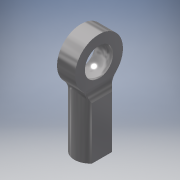
# Autodesk Inventor part: 10-32SuperDutyLinkage-1111-2017
Saved by Autodesk Inventor 2016 SP2 (Build 200236200, 236)
## iProperties
Created: 2017-02-16
Part Number: 10-32SuperDutyLinkage-1111-2017
Material: Stainless Steel
Document SubType Name: Modeling
Designer: 589013
Density: 8 g/cm^3
Appearance: Semi-Polished
Mass: 11.5391 g
Surface Area: 17.147 cm^2
Volume: 1.44239 cm^3
Author: 589013
Autodesk Inventor part; units mm, degrees
ref_plane "YZ Plane" through (0, 0, 0) normal (1, 0, 0) x (0, 1, 0)
ref_plane "XZ Plane" through (0, 0, 0) normal (0, 1, 0) x (-1, 0, 0)
ref_plane "XY Plane" through (0, 0, 0) normal (0, 0, 1) x (1, 0, 0)
sketch "Sketch1" plane through (0, 0, 0) normal (1, 0, 0) x (0, 1, 0)
  circle A0 centre (0, 0) radius 7.9375
  arc A1 (0, 5.55625) -> (0, -5.55625) centre (0, 0) ccw
  circle A2 centre (0, 0) radius 5.159375 construction
  line L0 (0, 5.159375) -> (0, -5.159375) construction
  line L1 (0, -5.159375) -> (-6.031978, -5.159375) construction
  line L2 (-26.9875, -5.159375) -> (-26.9875, 0)
  line L3 (-26.9875, 5.159375) -> (-6.031978, 5.159375) construction
  line L4 (-6.031978, 5.159375) -> (0, 5.159375) construction
  line L5 (-6.031978, -5.159375) -> (-26.9875, -5.159375)
  line L6 (-7.9375, 5.159375) -> (-7.9375, 0) construction
  line L7 (-7.9375, 0) -> (-26.9875, 0)
  line L8 (-26.9875, 0) -> (-26.9875, 5.159375) construction
  line L9 (-7.9375, 0) -> (-7.9375, -5.159375)
  line L10 (0, 5.55625) -> (0, -5.55625)
  arc A3 (0, -5.55625) -> (0, 5.55625) centre (0, 0) ccw construction
  dimension "d0" = 15.875
  dimension "d1" = 11.1125
  dimension "d2" = 10.31875
  dimension "d3" = 26.9875
  constraints: 22 end point, 9 point on circle, 6 parallel, 4 centre point, 4 perpendicular, 4 point on line, 3 coincident
  measures "d0" diameter of A0
  measures "d1" diameter of A1
  measures "d2" diameter of A2
  measures "d3" distance of L0.end L2.start
revolve "Revolution1" add sketch "Sketch1" angle 360 about axis through (0, -7.9375, 0) along (0, -1, 0) contours L9 L5 L2 L7
extrude "Extrusion1" add sketch "Sketch1" along normal mid plane 5.953125 contours A0 | L10 A1
revolve "Revolution2" cut sketch "Sketch1" angle 360 about axis through (0, 0, 5.55625) along (0, 0, -1) contours L10 A1
sketch "Sketch2" plane through (0, -7.9375, 0) normal (0, 1, 0) x (1, 0, 0)
  line L0 (-2.976562, 0) -> (2.976562, 0)
  circle A0 centre (0, 0) radius 5.159375
  point P0 (0, 0)
extrude "Extrusion2" add sketch "Sketch2" along normal up to surface round surface about axis through (0, 0, 0) along (1, 0, 0) radius 7.9375 far side no
fillet "Fillet1" radius 3.175 2 edges at (0, -6.032, 5.1594) (0, -6.032, -5.1594)
sketch "Sketch3" plane through (0, 0, 0) normal (0, 0, 1) x (1, 0, 0)
  arc A0 (2.976562, 4.691694) -> (-2.976562, 4.691694) centre (0, 0) ccw
  line L0 (-2.976562, 4.691694) -> (-2.976562, 7.9375)
  line L1 (-2.976562, 7.9375) -> (2.976562, 7.9375)
  line L2 (2.976562, 7.9375) -> (2.976562, 4.691694)
  arc A1 (-2.976562, -4.691694) -> (2.976562, -4.691694) centre (0, 0) ccw
  line L3 (2.976562, -4.691694) -> (2.976562, -7.9375)
  line L4 (2.976562, -7.9375) -> (5.159375, -7.9375)
  line L5 (5.159375, -7.9375) -> (5.159375, -26.9875)
  line L6 (5.159375, -26.9875) -> (-5.159375, -26.9875) construction
  line L7 (-5.159375, -26.9875) -> (-5.159375, -7.9375)
  line L8 (-5.159375, -7.9375) -> (-2.976562, -7.9375)
  line L9 (-2.976562, -7.9375) -> (-2.976562, -4.691694)
  line L10 (5.159375, -7.9375) -> (2.976562, -7.9375)
  line L11 (5.159375, -7.9375) -> (5.159375, -26.9875)
  line L12 (5.159375, -7.9375) -> (5.159375, -26.9875)
  line L13 (-2.976562, -7.9375) -> (-5.159375, -7.9375)
  line L14 (-5.159375, -7.9375) -> (-5.159375, -26.9875)
  line L15 (-5.159375, -7.9375) -> (-5.159375, -26.9875)
  line L16 (2.976562, -7.9375) -> (5.159375, -11.7475)
  line L17 (-2.976562, -7.9375) -> (-5.159375, -11.7475)
  line L18 (2.976562, -7.9375) -> (5.159375, -7.9375)
  line L19 (5.159375, -7.9375) -> (5.159375, -5.047949)
  line L20 (5.159375, -5.047949) -> (2.976562, -5.047949)
  line L21 (2.976562, -5.047949) -> (2.976562, -7.9375)
  line L22 (-2.976562, -7.9375) -> (-5.159375, -7.9375)
  line L23 (-5.159375, -7.9375) -> (-5.159375, -4.517345)
  line L24 (-5.159375, -4.517345) -> (-2.976562, -4.517345)
  line L25 (-2.976562, -4.517345) -> (-2.976562, -7.9375)
  dimension "d11" = 3.81
  dimension "d12" = 3.81
  constraints: 28 end point, 7 equal length, 2 collinear, 2 horizontal, 2 perpendicular, 2 point on line
  measures "d11" vertical distance of L8.end L17.end
  measures "d12" vertical distance of L3.end L16.end
extrude "Extrusion3" cut sketch "Sketch3" along normal through all both and the other way through all contours L20 L19 L4 L3 | L4 L5 L16 | L7 L8 L17 | L23 L24 L25 L9 L8
fillet "Fillet2" radius 6.35 4 edges at (-2.9766, -7.9375, 2.1071) (-2.9766, -7.9375, -2.1071) (2.9766, -7.9375, 2.1071) (2.9766, -7.9375, -2.1071)
hole "Hole1" at (0, -26.9875, 0) direction (0, 1, 0) diameter 7.9375 depth 12.7
thread "Thread1" size "5/16-18 UNC" class "2B" standard "ANSI Unified Screw Threads" full length
sketch "Sketch4" plane through (0, -26.9875, 0) normal (0, -1, 0) x (1, 0, 0)
  circle A0 centre (0, 0) radius 3.96875
  circle A1 centre (0, 0) radius 5.159375
  line L0 (-3.96875, 5.159375) -> (3.96875, 5.159375)
  line L1 (3.96875, 5.159375) -> (3.96875, -5.159375)
  line L2 (3.96875, -5.159375) -> (-3.96875, -5.159375)
  line L3 (-3.96875, -5.159375) -> (-3.96875, 5.159375)
  line L4 (-3.96875, 5.159375) -> (3.96875, -5.159375) construction
  line L5 (3.96875, 5.159375) -> (-3.96875, -5.159375) construction
  arc A2 (3.96875, -5.159375) -> (3.96875, 5.159375) centre (3.96875, 0) ccw
  arc A3 (-3.96875, 5.159375) -> (-3.96875, -5.159375) centre (-3.96875, 0) ccw
  line L6 (3.96875, 5.159375) -> (3.96875, -5.159375)
  point P0 (0, 0)
  point P1 (0, -5.159375)
  dimension "d27" = 7.9375
  constraints: 14 end point, 4 point on circle, 3 equal length, 3 midpoint, 3 tangent, 2 centre point, 1 horizontal, 1 perpendicular, 1 vertical alignment, 1 other
  measures "d27" distance of L1.end L2.end
extrude "Extrusion4" cut sketch "Sketch4" against normal through all contours L1 A1 | L3 A1 | L1 A2 A1 | L3 A3 A1
body "Solid1"
